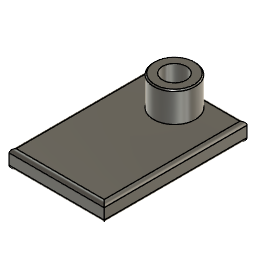
Prensa Mecánica Manual tipo leva (Ensamblaje) (1) (Autodesk Fusion 360 archive; units mm, degrees)
design "Es_Base"
part number: 2026-08-25-09-09-24-307
Autodesk Fusion 360 part; units mm, degrees
sketch "Boceto1" plane through (0, 0, 0) normal (0, 0, 1) x (1, 0, 0)
  line L0 (-40, 60) -> (40, 60)
  line L1 (40, 60) -> (40, -60)
  line L2 (40, -60) -> (-40, -60)
  line L3 (-40, -60) -> (-40, 60)
  line L4 (-40, 60) -> (40, -60) construction
  line L5 (40, 60) -> (-40, -60) construction
  constraint horizontal L0
  constraint perpendicular L0 L1
  constraint parallel L0 L2
  constraint parallel L1 L3
  constraint coincident L4 origin
  constraint coincident L5 origin
extrude "Extruir1" add sketch "Boceto1" along normal blind 15
fillet "Empalme1" radius 3 4 edges at (40, 0, 15) (0, -60, 15) (0, 60, 15) (-40, 0, 15) 1 faces at (-13.3333, 20, 0)
sketch "Boceto2" plane through (0, 0, 15) normal (0, 0, 1) x (-1, 0, 0)
  line L0 (37, -57) -> (37, 57)
  line L1 (37, 57) -> (-37, 57)
  line L2 (-37, 57) -> (-37, -57)
  line L3 (-37, -57) -> (37, -57)
  circle A0 centre (0.3597, -39.378) radius 17.5
  dimension "d5" = 35
  measures "d5" diameter of A0
extrude "Extruir2" add sketch "Boceto2" along normal blind 25 contours A0
sketch "Boceto3" plane through (0, 0, 40) normal (0, 0, 1) x (-1, 0, 0)
  circle A0 centre (0.3597, -39.378) radius 17.5
  circle A1 centre (0.3597, -39.378) radius 10
  dimension "d8" = 20
  constraint concentric A0 A1
  measures "d8" diameter of A1
extrude "Extruir3" cut sketch "Boceto3" against normal through all contours A1
chamfer "Chaflán1" distance 1 angle 45 1 edges at (15.956, 45.7063, 40)

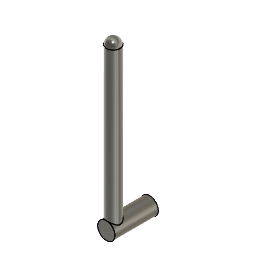
design "Brazo_movil"
part number: 2026-08-25-11-39-10-312
Autodesk Fusion 360 part; units mm, degrees
sketch "Boceto2" plane through (0, 0, 0) normal (1, 0, 0) x (0, 1, 0)
  line L0 (0, 0) -> (25, 0)
  line L1 (25, 0) -> (25, 5)
  line L2 (25, 5) -> (0, 5)
  line L3 (0, 5) -> (0, 0)
  dimension "d4" = 25
  dimension "d5" = 5
  constraint horizontal L0
  constraint vertical L1
  constraint horizontal L2
  constraint vertical L3
  constraint coincident L0.start L3.end
  measures "d4" distance of L0.start L0.end
  measures "d5" distance of L0.start L2.end
revolve "Revolución1" add sketch "Boceto2" angle 360 about axis through (0, 0, 0) along (0, 1, 0)
sketch "Boceto3" plane through (0, 0, 0) normal (0, 1, 0) x (1, 0, 0)
ref_plane "PlanoDeObra1" through (0, 0, 5) normal (0, 0, 1) x (1, 0, 0)
sketch "Boceto4" plane through (0, 0, 5) normal (0, 0, 1) x (1, 0, 0)
  circle A0 centre (0, 4) radius 4
  dimension "d9" = 8
  measures "d9" diameter of A0
extrude "Extruir2" add sketch "Boceto4" along normal blind 90 and the other way blind 2
fillet "Empalme1" radius 4 1 faces at (1.2741, 3.9956, 95)

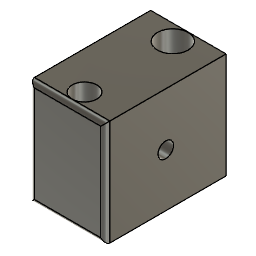
design "Cabezal"
part number: 2026-08-25-09-55-48-521
Autodesk Fusion 360 part; units mm, degrees
sketch "Boceto1" plane through (0, 0, 0) normal (0, 1, 0) x (1, 0, 0)
  line L0 (25, 35) -> (-25, 35)
  line L1 (-25, 35) -> (-25, -35)
  line L2 (-25, -35) -> (25, -35)
  line L3 (25, -35) -> (25, 35)
  line L4 (25, 35) -> (-25, -35) construction
  line L5 (-25, 35) -> (25, -35) construction
  dimension "d1" = 50
  dimension "d2" = 70
  constraint horizontal L0
  constraint perpendicular L0 L1
  constraint parallel L0 L2
  constraint parallel L1 L3
  constraint coincident L4 origin
  constraint coincident L5 origin
  measures "d1" distance of L1.end L2.end
  measures "d2" distance of L0.end L1.end
extrude "Extruir1" add sketch "Boceto1" along normal mid plane 80
fillet "Empalme1" radius 3 4 edges at (25, -40, 0) (-25, -40, 0) (0, -40, 35) (0, -40, -35) 1 faces at (-8.3333, -40, -11.6667)
sketch "Boceto2" plane through (0, 0, 35) normal (0, 0, 1) x (-1, 0, 0)
  line L0 (25, 37) -> (-25, 37)
  line L1 (-25, 37) -> (-25, -40)
  line L2 (-25, -40) -> (25, -40)
  line L3 (25, -40) -> (25, 37)
  circle A0 centre (0.02, -29.7568) radius 10.15
  circle A1 centre (0.0305, 28.7522) radius 8.15
  dimension "d7" = 20.3
  dimension "d8" = 16.3
  measures "d7" diameter of A0
  measures "d8" diameter of A1
extrude "Extruir2" cut sketch "Boceto2" along normal through all and the other way through all contours A1
sketch "Boceto3" plane through (0, 0, 35) normal (0, 0, 1) x (-1, 0, 0)
  circle A0 centre (0.0305, 28.7522) radius 8.15
  line L0 (25, 37) -> (-25, 37)
  line L1 (-25, 37) -> (-25, -40)
  line L2 (-25, -40) -> (25, -40)
  line L3 (25, -40) -> (25, 37)
  circle A1 centre (-0.0995, -29.5564) radius 10.15
  dimension "d10" = 20.3
  measures "d10" diameter of A1
extrude "Extruir3" cut sketch "Boceto3" along normal through all and the other way through all contours A1
sketch "Boceto4" plane through (25, 0, 0) normal (1, 0, 0) x (0, 1, 0)
  line L0 (-37, 35) -> (-37, -35)
  line L1 (-37, -35) -> (40, -35)
  line L2 (40, -35) -> (40, 35)
  line L3 (40, 35) -> (-37, 35)
  circle A0 centre (0, 0) radius 5.15
  dimension "d12" = 10.3
  constraint coincident A0.centre origin
  measures "d12" diameter of A0
extrude "Extruir4" cut sketch "Boceto4" against normal through all contours A0

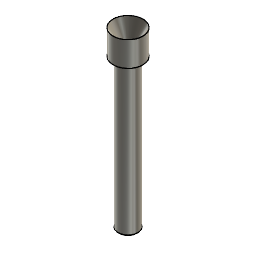
design "piston"
part number: 2026-08-25-10-17-09-336
Autodesk Fusion 360 part; units mm, degrees
sketch "Boceto1" plane through (0, 0, 0) normal (0, 1, 0) x (1, 0, 0)
  line L0 (0, 0) -> (0, -120)
  line L1 (0, 0) -> (8, 0)
  line L2 (8, 0) -> (8, -120)
  line L3 (8, -120) -> (12, -120)
  line L4 (12, -120) -> (12, -140)
  line L5 (12, -140) -> (0, -120)
  dimension "d1" = 120
  dimension "d2" = 8
  dimension "d3" = 120
  dimension "d4" = 4
  dimension "d5" = 20
  constraint coincident L0.start L1.start
  constraint vertical L0
  constraint perpendicular L0 L1
  constraint perpendicular L1 L2
  constraint perpendicular L2 L3
  constraint perpendicular L3 L4
  measures "d1" distance of L0.start L0.end
  measures "d2" distance of L0.start L1.end
  measures "d3" distance of L1.end L2.end
  measures "d4" distance of L2.end L3.end
  measures "d5" distance of L3.end L4.end
revolve "Revolución1" add sketch "Boceto1" angle 360 about axis through (0, 0, 0) along (0, 0, 1)
chamfer "Chaflán1" distance 1 angle 45 1 edges at (-7.4586, -2.8929, 0)
